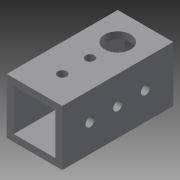
# Autodesk Inventor part: 2 in 3-8 in Hex Shaft Holders (4)
Saved by Autodesk Inventor 2014 (Build 180170000, 170)
## iProperties
Created: 2014-02-24
Part Number: 2 in 3-8 in Hex Shaft Holders (4)
Material: Generic
Document SubType Name: Modeling
Designer: Michael
Density: 1 g/cm^3
Appearance: Default
Author: Michael
Autodesk Inventor part; units mm, degrees
ref_plane "YZ Plane" through (0, 0, 0) normal (1, 0, 0) x (0, 1, 0)
ref_plane "XZ Plane" through (0, 0, 0) normal (0, 1, 0) x (-1, 0, 0)
ref_plane "XY Plane" through (0, 0, 0) normal (0, 0, 1) x (1, 0, 0)
sketch "Sketch1" plane through (0, 0, 0) normal (0, 0, 1) x (1, 0, 0)
  line L0 (0, 0) -> (25.4, 0)
  line L1 (25.4, 0) -> (25.4, 25.4)
  line L2 (25.4, 25.4) -> (0, 25.4)
  line L3 (0, 25.4) -> (0, 0)
  line L4 (3.175, 22.225) -> (22.225, 22.225)
  line L5 (22.225, 22.225) -> (22.225, 3.175)
  line L6 (22.225, 3.175) -> (3.175, 3.175)
  line L7 (3.175, 3.175) -> (3.175, 22.225)
  dimension "d0" = 25.4
  dimension "d1" = 25.4
  dimension "d2" = 3.175
  constraints: 16 end point, 4 parallel, 2 perpendicular, 1 horizontal, 3 other
  measures "d0" distance of L2.end L1.end
  measures "d1" distance of L1.end L0.end
  measures "d2" distance between parallel lines of L4 L2
extrude "Extrusion1" add sketch "Sketch1" along normal blind 50.8
sketch "Sketch2" plane through (25.4, 0, 0) normal (1, 0, 0) x (0, 0, -1)
  line L0 (-50.8, 0) -> (-50.8, 25.4) projected
  line L1 (0, 0) -> (-50.8, 0) projected
  circle A0 centre (-38.1, 12.7) radius 2.0701
  circle A1 centre (-25.4, 12.7) radius 2.0701
  circle A2 centre (-12.7, 12.7) radius 2.0701
  dimension "d5" = 4.1402
  dimension "d6" = 12.7
  dimension "d7" = 12.7
  dimension "d10" = 12.7
  constraints: 3 centre point, 1 horizontal, 4 other
  measures "d5" diameter of A0
  measures "d6" distance from line of L0 A0.centre
  measures "d7" distance from line of L1 A0.centre
  measures "d10" distance of A0.centre A1.centre
extrude "Extrusion2" cut sketch "Sketch2" against normal blind 50.8
sketch "Sketch3" plane through (0, 25.4, 0) normal (0, 1, 0) x (1, 0, 0)
  line L0 (25.4, -50.8) -> (0, -50.8) projected
  line L1 (25.4, 0) -> (25.4, -50.8) projected
  circle A0 centre (12.7, -38.1) radius 2.0701
  circle A1 centre (12.7, -25.4) radius 2.0701
  circle A2 centre (12.7, -12.7) radius 5.9531
  dimension "d17" = 4.1402
  dimension "d18" = 12.7
  dimension "d19" = 12.7
  dimension "d22" = 12.7
  dimension "d27" = 11.9062
  dimension "d28" = 12.7
  dimension "d29" = 12.7
  constraints: 3 centre point, 1 vertical, 2 other
  measures "d17" diameter of A0
  measures "d18" distance from line of L0 A0.centre
  measures "d19" distance from line of L1 A0.centre
  measures "d22" distance of A0.centre A1.centre
  measures "d27" diameter of A2
  measures "d28" distance of A2.centre A1.centre
  measures "d29" distance from line of A2.centre L1
extrude "Extrusion3" cut sketch "Sketch3" against normal blind 50.8
body "Solid1"
